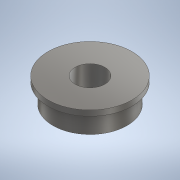
# Autodesk Inventor part: ベアリング 6.15
Saved by Autodesk Inventor 2020 (Build 240168000, 168)
## iProperties
Part Number: ベアリング 6.15
Material: ステンレス鋼
Document SubType Name: Modeling
Designer: 原知也
Density: 8 g/cm^3
Appearance: 半つや出し
Mass: 6.26119 g
Surface Area: 7.27593 cm^2
Volume: 0.782649 cm^3
Author: 原知也
Autodesk Inventor part; units mm, degrees
ref_plane "YZ Plane" through (0, 0, 0) normal (1, 0, 0) x (0, 1, 0)
ref_plane "XZ Plane" through (0, 0, 0) normal (0, 1, 0) x (-1, 0, 0)
ref_plane "XY Plane" through (0, 0, 0) normal (0, 0, 1) x (1, 0, 0)
sketch "スケッチ1" plane through (0, 0, 0) normal (0, 0, 1) x (1, 0, 0)
  circle A0 centre (0, 0) radius 3
  circle A1 centre (0, 0) radius 7.5
  dimension "d0" = 6
  dimension "d1" = 15
  constraints: 2 centre point, 2 coincident
  measures "d0" diameter of A0
  measures "d1" diameter of A1
extrude "押し出し1" add sketch "スケッチ1" along normal blind 3.9
sketch "スケッチ2" plane through (0, 0, 3.9) normal (0, 0, 1) x (1, 0, 0)
  circle A0 centre (0, 0) radius 8.5
  circle A1 centre (0, 0) radius 3
  dimension "d4" = 17
  dimension "d5" = 6
  constraints: 2 centre point, 2 coincident
  measures "d4" diameter of A0
  measures "d5" diameter of A1
extrude "押し出し2" add sketch "スケッチ2" along normal blind 1.1
